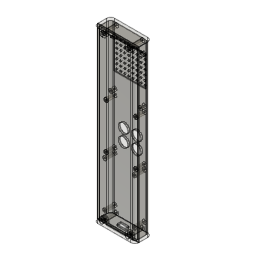
remote (Autodesk Fusion 360 design; units mm, degrees)
part number: 2025-07-19-14-33-31-747
part number: 2025-07-19-16-18-06-668
Autodesk Fusion 360 part; units mm, degrees
sketch "end" plane through (0, 0, 0) normal (0, 0, 1) x (1, 0, 0)
  line L0 (-20, 10) -> (21, 10)
  line L1 (26, 5) -> (26, -6)
  line L2 (21, -11) -> (-20, -11)
  line L3 (-25, -6) -> (-25, 5)
  arc A0 (-20, 10) -> (-25, 5) centre (-20, 5) ccw
  arc A1 (-25, -6) -> (-20, -11) centre (-20, -6) ccw
  arc A2 (26, 5) -> (21, 10) centre (21, 5) ccw
  arc A3 (21, -11) -> (26, -6) centre (21, -6) ccw
  arc A4 (24, 5) -> (21, 8) centre (21, 5) ccw
  line L4 (-20, 8) -> (21, 8)
  arc A5 (-20, 8) -> (-23, 5) centre (-20, 5) ccw
  line L5 (-23, -6) -> (-23, 5)
  arc A6 (-23, -6) -> (-20, -9) centre (-20, -6) ccw
  line L6 (21, -9) -> (-20, -9)
  arc A7 (21, -9) -> (24, -6) centre (21, -6) ccw
  line L7 (24, 5) -> (24, -6)
  point P0 (-25, 10)
  point P1 (26, 10)
  point P2 (-25, -11)
  dimension "d1" = 51
  dimension "d2" = 21
  dimension "d3" = 5
  dimension "d4" = 5
  dimension "d5" = 5
  dimension "d6" = 5
  dimension "d7" = 2
  constraint horizontal L0
  constraint vertical L1
  constraint horizontal L2
  constraint vertical L3
  constraint coincident P0 L0
  constraint coincident P0 L3
  constraint tangent L0 A0
  constraint tangent L3 A0
  constraint coincident P2 L2
  constraint coincident P2 L3
  constraint tangent L2 A1
  constraint tangent L3 A1
  constraint coincident P1 L0
  constraint coincident P1 L1
  constraint tangent L0 A2
  constraint tangent L1 A2
  constraint tangent L1 A3
  constraint tangent L2 A3
  measures "d1" distance of P0 P1
  measures "d2" distance of P0 P2
  measures "d3" radius of A0 P2
  measures "d4" radius of A1 P2
  measures "d5" radius of A2
  measures "d6" radius of A3
extrude "Extrude1" add sketch "end" along normal blind 202 makes body 1
sketch "wall" plane through (0, 0, 0) normal (0, 0, 1) x (1, 0, 0)
  line L0 (21, -11) -> (-20, -11)
  arc A0 (-20, 10) -> (-25, 5) centre (-20, 5) ccw
  line L1 (-20, 10) -> (21, 10)
  arc A1 (-25, -6) -> (-20, -11) centre (-20, -6) ccw
  line L2 (-25, -6) -> (-25, 5)
  arc A2 (21, -11) -> (26, -6) centre (21, -6) ccw
  arc A3 (26, 5) -> (21, 10) centre (21, 5) ccw
  line L3 (26, 5) -> (26, -6)
  point P0 (26, 10)
  point P1 (-25, 10)
  point P2 (-25, -11)
  dimension "d10" = 51
  dimension "d11" = 21
  dimension "d12" = 5
  dimension "d13" = 5
  dimension "d14" = 5
  dimension "d15" = 5
  constraint horizontal L1
  constraint vertical L3
  constraint horizontal L0
  constraint vertical L2
  constraint coincident P1 L1
  constraint coincident P1 L2
  constraint tangent A0 L1
  constraint tangent A0 L2
  constraint coincident P2 L0
  constraint coincident P2 L2
  constraint tangent L0 A1
  constraint tangent A1 L2
  constraint coincident P0 L1
  constraint coincident P0 L3
  constraint tangent L1 A3
  constraint tangent A3 L3
  constraint tangent A2 L3
  constraint tangent L0 A2
  measures "d10" distance of P0 P1
  measures "d11" distance of P1 P2
  measures "d12" radius of A0
  measures "d13" radius of A1
  measures "d14" radius of A3
  measures "d15" radius of A2
extrude "Extrude2" add sketch "end" along normal blind 2 separate body contours L0 L1 L2 L3 A0 A1 A2 A3 | A4 L4 A5 L5 A6 L6 A7 L7 makes body 2
copy_body "CopyPasteBodies1" bodies 2 makes body 3
move_body "Move1" bodies 3 to x (1, 0, 0) y (0, 1, 0) z (0, 0, 1) at (0, 0, 200)
cylinder "CylinderPrimitive3" add diameter 5 height 12.5 placed x (1, 0, 0) y (0, 0, -1) z (0, 1, 0) at (-55, 0, 80) separate body makes body 4
cylinder "CylinderPrimitive4" cut diameter 1.7 height -12.5 placed x (1, 0, 0) y (0, 0, 1) z (0, -1, 0) at (-55, 0, 80) bodies 4
move_body "Move2" bodies 4 to x (1, 0, 0) y (0, 1, 0) z (0, 0, 1) at (0, -4.5, 0)
move_body "Move3" bodies 4 to x (1, 0, 0) y (0, 1, 0) z (0, 0, 1) at (0, 0, -77.5)
move_body "Move4" bodies 4 to x (1, 0, 0) y (0, 1, 0) z (0, 0, 1) at (0, 0, 9.5)
move_body "Move5" bodies 4 to x (1, 0, 0) y (0, 1, 0) z (0, 0, 1) at (32.5, 0, 0)
copy_body "CopyPasteBodies2" bodies 4 makes body 5
move_body "Move6" bodies 5 to x (1, 0, 0) y (0, 1, 0) z (0, 0, 1) at (46, 0, 0)
move_body "Move7" bodies 4 to x (1, 0, 0) y (0, 1, 0) z (0, 0, 1) at (4.75, 0, 0)
move_body "Move8" bodies 5 to x (1, 0, 0) y (0, 1, 0) z (0, 0, 1) at (-4.75, 0, 0)
copy_body "CopyPasteBodies3" bodies 4 makes body 6
move_body "Move9" bodies 6 to x (1, 0, 0) y (0, 1, 0) z (0, 0, 1) at (0, 0, 56)
copy_body "CopyPasteBodies4" bodies 5 makes body 7
move_body "Move10" bodies 7 to x (1, 0, 0) y (0, 1, 0) z (0, 0, 1) at (0, 0, 56)
cylinder "CylinderPrimitive5" add diameter 5 height 10.2 placed x (1, 0, 0) y (0, 0, -1) z (0, 1, 0) at (50, 10, 10) separate body makes body 8
cylinder "CylinderPrimitive6" cut diameter 1.7 height 10.2 placed x (1, 0, 0) y (0, 0, -1) z (0, 1, 0) at (50, 10, 10) bodies 8
move_body "Move11" bodies 8 to x (1, 0, 0) y (0, 1, 0) z (0, 0, 1) at (-26.5, 0, 0)
move_body "Move12" bodies 8 to x (1, 0, 0) y (0, 1, 0) z (0, 0, 1) at (0, -12.2, 0)
copy_body "CopyPasteBodies5" bodies 8 makes body 9
move_body "Move13" bodies 9 to x (1, 0, 0) y (0, 1, 0) z (0, 0, 1) at (-46, 0, 0)
move_body "Move14" bodies 8 to x (1, 0, 0) y (0, 1, 0) z (0, 0, 1) at (-4.7, 0, 0)
move_body "Move15" bodies 9 to x (1, 0, 0) y (0, 1, 0) z (0, 0, 1) at (4.7, 0, 0)
move_body "Move16" bodies 8 9 to x (1, 0, 0) y (0, 1, 0) z (0, 0, 1) at (0, 0, -7.5)
move_body "Move17" bodies 8 9 to x (1, 0, 0) y (0, 1, 0) z (0, 0, 1) at (0, 0, 71.2)
copy_body "CopyPasteBodies6" bodies 8 9 makes body 10 makes body 11
move_body "Move18" bodies 10 11 to x (1, 0, 0) y (0, 1, 0) z (0, 0, 1) at (0, 0, 56)
cylinder "CylinderPrimitive7" add diameter 5 height 5 placed x (1, 0, 0) y (0, 0, -1) z (0, 1, 0) at (35, 0, 115) separate body makes body 12
cylinder "CylinderPrimitive8" cut diameter 1.7 height 5 placed x (1, 0, 0) y (0, 0, -1) z (0, 1, 0) at (35, 0, 115) bodies 12
move_body "Move19" bodies 12 to x (1, 0, 0) y (0, 1, 0) z (0, 0, 1) at (-11.5, 0, 84.5)
copy_body "CopyPasteBodies7" bodies 12 makes body 13
move_body "Move20" bodies 13 to x (1, 0, 0) y (0, 1, 0) z (0, 0, 1) at (-46, 0, 0)
move_body "Move21" bodies 12 to x (1, 0, 0) y (0, 1, 0) z (0, 0, 1) at (-4.7, 0, 0)
move_body "Move22" bodies 13 to x (1, 0, 0) y (0, 1, 0) z (0, 0, 1) at (4.7, 0, 0)
move_body "Move23" bodies 12 13 to x (1, 0, 0) y (0, 1, 0) z (0, 0, 1) at (0, 0, -7.1)
copy_body "CopyPasteBodies8" bodies 12 13 makes body 14 makes body 15
move_body "Move24" bodies 14 15 to x (1, 0, 0) y (0, 1, 0) z (0, 0, 1) at (0, 0, -56)
move_body "Move25" bodies 12 13 14 15 to x (1, 0, 0) y (0, 1, 0) z (0, 0, 1) at (0, 3, 0)
ref_plane "WorkPlane1" through (0, -6, 0) normal (0, 1, 0) x (0, 0, 1)
combine "Combine1" operation add target body 1 tool bodies 3 5 2 4 7 6 9 8 10 12 11 13 14 15 keep tools result as body 16 in component "Component"
split "Split1" by plane through (0, -6, 0) normal (0, 1, 0) bodies 16 makes body 17 at (-6.3333, 10, 134.6667) in component "Component"
cylinder "CylinderPrimitive9" add diameter 5 height 14 placed x (1, 0, 0) y (0, 0, -1) z (0, 1, 0) at (50, 0, 50) separate body makes body 18
cylinder "CylinderPrimitive10" cut diameter 1.7 height 14 placed x (1, 0, 0) y (0, 0, -1) z (0, 1, 0) at (50, 0, 50) bodies 18
move_body "Move26" bodies 18 to x (1, 0, 0) y (0, 1, 0) z (0, 0, 1) at (-26.5, 0, 0)
move_body "Move27" bodies 18 to x (1, 0, 0) y (0, 1, 0) z (0, 0, 1) at (0, 0, -47.5)
copy_body "CopyPasteBodies9" bodies 18 makes body 19
move_body "Move28" bodies 19 to x (1, 0, 0) y (0, 1, 0) z (0, 0, 1) at (-46, 0, 0)
move_body "Move29" bodies 18 to x (1, 0, 0) y (0, 1, 0) z (0, 0, 1) at (-7, 0, 2)
move_body "Move30" bodies 19 to x (1, 0, 0) y (0, 1, 0) z (0, 0, 1) at (7, 0, 2)
move_body "Move31" bodies 18 19 to x (1, 0, 0) y (0, 1, 0) z (0, 0, 1) at (0, -6, 0)
move_body "Move32" bodies 18 19 to x (1, 0, 0) y (0, 1, 0) z (0, 0, 1) at (0, 0, 193)
combine "Combine2" operation add target body 17 tool bodies 18 19 keep tools in component "Component"
cylinder "CylinderPrimitive11" add diameter 5 height 5 placed x (1, 0, 0) y (0, 0, -1) z (0, 1, 0) at (35, 0, 165) separate body makes body 20
move_body "Move33" bodies 20 to x (1, 0, 0) y (0, 1, 0) z (0, 0, 1) at (0, -12, 32.5)
move_body "Move34" bodies 20 to x (1, 0, 0) y (0, 1, 0) z (0, 0, 1) at (-50.5, 0, 0)
combine "Combine3" operation cut target body 16 tool bodies 20 keep tools in component "Component"
move_body "Move35" bodies 20 to x (1, 0, 0) y (0, 1, 0) z (0, 0, 1) at (32, 0, 0)
combine "Combine4" operation cut target body 16 tool bodies 20 keep tools in component "Component"
move_body "Move36" bodies 20 to x (1, 0, 0) y (0, 1, 0) z (0, 0, 1) at (0, 0, -193)
copy_body "CopyPasteBodies10" bodies 18 19 makes body 21 makes body 22
move_body "Move37" bodies 21 22 to x (1, 0, 0) y (0, 1, 0) z (0, 0, 1) at (0, 0, -193)
combine "Combine5" operation add target body 17 tool bodies 21 22 keep tools in component "Component"
combine "Combine6" operation cut target body 16 tool bodies 20 keep tools in component "Component"
move_body "Move38" bodies 20 to x (1, 0, 0) y (0, 1, 0) z (0, 0, 1) at (-32, 0, 0)
combine "Combine7" operation cut target body 16 tool bodies 20 keep tools in component "Component"
cylinder "CylinderPrimitive12" add diameter 9 height 5 placed x (1, 0, 0) y (0, 0, -1) z (0, 1, 0) at (40, 0, 5) separate body makes body 23
cylinder "CylinderPrimitive13" add diameter 5 height 3 placed x (1, 0, 0) y (0, 0, -1) z (0, 1, 0) at (40, 0, 15) separate body makes body 24
move_body "Move39" bodies 24 to x (1, 0, 0) y (0, 1, 0) z (0, 0, 1) at (0, 0, -10)
combine "Combine1'" operation cut target body 23 tool bodies 24
cylinder "CylinderPrimitive14" add diameter 2 height 5 placed x (1, 0, 0) y (0, 0, -1) z (0, 1, 0) at (50, 0, 5) separate body makes body 25
move_body "Move40" bodies 25 to x (1, 0, 0) y (0, 1, 0) z (0, 0, 1) at (-10, 0, 0)
combine "Combine2'" operation cut target body 23 tool bodies 25
move_body "Move41" bodies 23 to x (1, 0, 0) y (0, 1, 0) z (0, 0, 1) at (-23.5, -11, 0)
move_body "Move42" bodies 23 to x (1, 0, 0) y (0, 1, 0) z (0, 0, 1) at (0, 0, -0.5)
copy_body "CopyPasteBodies11" bodies 23 makes body 26
move_body "Move43" bodies 26 to x (1, 0, 0) y (0, 1, 0) z (0, 0, 1) at (-32, 0, 0)
copy_body "CopyPasteBodies12" bodies 23 26 makes body 27 makes body 28
move_body "Move44" bodies 27 28 to x (1, 0, 0) y (0, 1, 0) z (0, 0, 1) at (0, 0, 193)
combine "Combine8" operation add target body 16 tool bodies 23 26 27 28 keep tools in component "Component"
cylinder "CylinderPrimitive15" add diameter 12 height 3 placed x (1, 0, 0) y (0, 0, -1) z (0, 1, 0) at (-50, 0, 50) separate body makes body 29
move_body "Move45" bodies 29 to x (1, 0, 0) y (0, 1, 0) z (0, 0, 1) at (0, 7.5, 0)
move_body "Move46" bodies 29 to x (1, 0, 0) y (0, 1, 0) z (0, 0, 1) at (70, 0, 34)
move_body "Move47" bodies 29 to x (1, 0, 0) y (0, 1, 0) z (0, 0, 1) at (-11.5, 0, 0)
copy_body "CopyPasteBodies13" bodies 29 makes body 30
move_body "Move48" bodies 30 to x (1, 0, 0) y (0, 1, 0) z (0, 0, 1) at (-27.5, 0, 0)
move_body "Move49" bodies 30 to x (1, 0, 0) y (0, 1, 0) z (0, 0, 1) at (11.5, 0, 0)
copy_body "CopyPasteBodies14" bodies 29 30 makes body 31 makes body 32
move_body "Move50" bodies 31 32 to x (1, 0, 0) y (0, 1, 0) z (0, 0, 1) at (0, 0, 14.8)
combine "Combine9" operation cut target body 17 tool bodies 29 30 31 32 keep tools in component "Component"
cylinder "CylinderPrimitive16" add diameter 2 height 5 placed x (1, 0, 0) y (0, 0, -1) z (0, 1, 0) at (82.0481, 0, 56.4909) separate body makes body 33
pattern_linear "R-Pattern1" count 8 spacing 5 along (1, 0, 0) count 10 spacing 5.5556 along (0, 0, 1) of bodies 33 makes body 34 at (87.9878, 1.6667, 56.1489) makes body 35 at (92.9878, 1.6667, 56.1489) makes body 36 at (97.9878, 1.6667, 56.1489) makes body 37 at (102.9878, 1.6667, 56.1489) makes body 38 at (107.9878, 1.6667, 56.1489) makes body 39 at (112.9878, 1.6667, 56.1489) makes body 40 at (117.9878, 1.6667, 56.1489) makes body 41 at (82.9878, 1.6667, 61.7044) makes body 42 at (87.9878, 1.6667, 61.7044) makes body 43 at (92.9878, 1.6667, 61.7044) makes body 44 at (97.9878, 1.6667, 61.7044) makes body 45 at (102.9878, 1.6667, 61.7044) makes body 46 at (107.9878, 1.6667, 61.7044) makes body 47 at (112.9878, 1.6667, 61.7044) makes body 48 at (117.9878, 1.6667, 61.7044) makes body 49 at (81.079, 1.6667, 67.3552) makes body 50 at (86.079, 1.6667, 67.3552) makes body 51 at (91.079, 1.6667, 67.3552) makes body 52 at (96.079, 1.6667, 67.3552) makes body 53 at (101.079, 1.6667, 67.3552) makes body 54 at (106.079, 1.6667, 67.3552) makes body 55 at (111.079, 1.6667, 67.3552) makes body 56 at (116.079, 1.6667, 67.3552) makes body 57 at (81.079, 1.6667, 72.9108) makes body 58 at (86.079, 1.6667, 72.9108) makes body 59 at (91.079, 1.6667, 72.9108) makes body 60 at (96.079, 1.6667, 72.9108) makes body 61 at (101.079, 1.6667, 72.9108) makes body 62 at (106.079, 1.6667, 72.9108) makes body 63 at (111.079, 1.6667, 72.9108) makes body 64 at (116.079, 1.6667, 72.9108) makes body 65 at (81.079, 1.6667, 78.4663) makes body 66 at (86.079, 1.6667, 78.4663) makes body 67 at (91.079, 1.6667, 78.4663) makes body 68 at (96.079, 1.6667, 78.4663) makes body 69 at (101.079, 1.6667, 78.4663) makes body 70 at (106.079, 1.6667, 78.4663) makes body 71 at (111.079, 1.6667, 78.4663) makes body 72 at (116.079, 1.6667, 78.4663) makes body 73 at (81.079, 1.6667, 84.0219) makes body 74 at (86.079, 1.6667, 84.0219) makes body 75 at (91.079, 1.6667, 84.0219) makes body 76 at (96.079, 1.6667, 84.0219) makes body 77 at (101.079, 1.6667, 84.0219) makes body 78 at (106.079, 1.6667, 84.0219) makes body 79 at (111.079, 1.6667, 84.0219) makes body 80 at (116.079, 1.6667, 84.0219) makes body 81 at (81.079, 1.6667, 89.5775) makes body 82 at (86.079, 1.6667, 89.5775) makes body 83 at (91.079, 1.6667, 89.5775) makes body 84 at (96.079, 1.6667, 89.5775) makes body 85 at (101.079, 1.6667, 89.5775) makes body 86 at (106.079, 1.6667, 89.5775) makes body 87 at (111.079, 1.6667, 89.5775) makes body 88 at (116.079, 1.6667, 89.5775) makes body 89 at (81.079, 1.6667, 95.133) makes body 90 at (86.079, 1.6667, 95.133) makes body 91 at (91.079, 1.6667, 95.133) makes body 92 at (96.079, 1.6667, 95.133) makes body 93 at (101.079, 1.6667, 95.133) makes body 94 at (106.079, 1.6667, 95.133) makes body 95 at (111.079, 1.6667, 95.133) makes body 96 at (116.079, 1.6667, 95.133) makes body 97 at (81.079, 1.6667, 100.6886) makes body 98 at (86.079, 1.6667, 100.6886) makes body 99 at (91.079, 1.6667, 100.6886) makes body 100 at (96.079, 1.6667, 100.6886) makes body 101 at (101.079, 1.6667, 100.6886) makes body 102 at (106.079, 1.6667, 100.6886) makes body 103 at (111.079, 1.6667, 100.6886) makes body 104 at (116.079, 1.6667, 100.6886) makes body 105 at (81.079, 1.6667, 106.2441) makes body 106 at (86.079, 1.6667, 106.2441) makes body 107 at (91.079, 1.6667, 106.2441) makes body 108 at (96.079, 1.6667, 106.2441) makes body 109 at (101.079, 1.6667, 106.2441) makes body 110 at (106.079, 1.6667, 106.2441) makes body 111 at (111.079, 1.6667, 106.2441) makes body 112 at (116.079, 1.6667, 106.2441)
move_body "Move51" bodies 104 91 66 34 101 65 38 82 85 81 67 48 41 108 59 86 70 106 89 39 61 57 79 77 96 75 102 71 98 109 78 99 36 95 83 37 111 80 69 110 53 44 33 103 49 112 84 58 43 52 51 45 76 50 42 62 88 100 107 105 40 46 73 64 97 47 92 72 55 54 87 35 63 93 68 56 74 94 60 90 to x (1, 0, 0) y (0, 1, 0) z (0, 0, 1) at (-99, 0, 84)
move_body "Move52" bodies 33 58 60 59 61 62 63 56 57 55 35 34 71 70 72 73 74 75 65 67 64 66 68 69 48 46 47 52 54 53 38 37 44 45 43 36 94 95 96 98 97 99 101 100 102 103 104 105 42 79 81 80 82 83 84 85 88 86 87 90 89 93 91 92 77 78 76 40 41 39 50 51 49 107 108 106 109 111 110 112 to x (1, 0, 0) y (0, 1, 0) z (0, 0, 1) at (0, -12, 0)
combine "Combine10" operation cut target body 17 tool bodies 33 58 60 59 61 62 63 56 57 55 35 34 71 70 72 73 74 75 65 67 64 66 68 69 48 46 47 52 54 53 38 37 44 45 43 36 94 95 96 98 97 99 101 100 102 103 104 105 42 79 81 80 82 83 84 85 88 86 87 90 89 93 91 92 77 78 76 40 41 39 50 51 49 107 108 106 109 111 110 112 keep tools in component "Component"
move_body "Move53" bodies 34 46 90 60 61 96 79 38 36 56 111 97 99 104 81 92 43 109 103 83 95 40 89 100 42 45 67 107 35 48 39 84 33 91 112 106 50 57 74 108 53 88 44 64 75 63 73 59 87 47 52 76 78 71 65 70 77 49 105 72 69 80 101 102 85 93 110 62 41 68 94 54 82 37 66 51 98 55 58 86 to x (1, 0, 0) y (0, 1, 0) z (0, 0, 1) at (0, 19, 0)
combine "Combine11" operation cut target body 17 tool bodies 33 58 60 59 61 62 63 56 57 55 35 34 71 70 72 73 74 75 65 67 64 66 68 69 48 46 47 52 54 53 38 37 44 45 43 36 94 95 96 98 97 99 101 100 102 103 104 105 42 79 81 80 82 83 84 85 88 86 87 90 89 93 91 92 77 78 76 40 41 39 50 51 49 107 108 106 109 111 110 112 keep tools in component "Component"
box "BoxPrimitive1" add length 5 width 10 height 4 placed x (0, 1, 0) y (-1, 0, 0) z (0, 0, 1) at (-1, 21, 0) separate body makes body 113
move_body "Move54" bodies 113 to x (1, 0, 0) y (0, 1, 0) z (0, 0, 1) at (0, -16, 0)
move_body "Move55" bodies 113 to x (1, 0, 0) y (0, 1, 0) z (0, 0, 1) at (-14, -6.5, 0)
move_body "Move56" bodies 113 to x (1, 0, 0) y (0, 1, 0) z (0, 0, 1) at (20.5, 0, 0)
move_body "Move57" bodies 113 to x (1, 0, 0) y (0, 1, 0) z (0, 0, 1) at (-1.27, 0, 0)
combine "Combine12" operation cut target body 17 tool bodies 113 keep tools in component "Component"
box "BoxPrimitive2" add length 6 width 43 height 2 placed x (0, 0, -1) y (-1, 0, 0) z (0, 1, 0) at (22, 0, 195) separate body makes body 114
move_body "Move58" bodies 114 to x (1, 0, 0) y (0, 1, 0) z (0, 0, 1) at (0, 3, 0)
combine "Combine13" operation cut target body 17 tool bodies 114 keep tools in component "Component"
cylinder "CylinderPrimitive17" add diameter 5 height 2 placed x (1, 0, 0) y (0, 0, -1) z (0, 1, 0) at (-15, 10, 130) separate body makes body 115
move_body "Move59" bodies 115 to x (1, 0, 0) y (0, 1, 0) z (0, 0, 1) at (-2.8, 0, -0.3)
cylinder "CylinderPrimitive18" add diameter 1.7 height 2 placed x (1, 0, 0) y (0, 0, -1) z (0, 1, 0) at (-20, 10, 139) separate body makes body 116
move_body "Move60" bodies 116 to x (1, 0, 0) y (0, 1, 0) z (0, 0, 1) at (2.2, 0, -2.6)
move_body "Move61" bodies 116 to x (1, 0, 0) y (0, 1, 0) z (0, 0, 1) at (0, 0, -6.7)
move_body "Move62" bodies 116 to x (1, 0, 0) y (0, 1, 0) z (0, 0, 1) at (0, -12.2, 0)
move_body "Move63" bodies 115 to x (1, 0, 0) y (0, 1, 0) z (0, 0, 1) at (0, -14.2, 0)
move_body "Move64" bodies 116 to x (1, 0, 0) y (0, 1, 0) z (0, 0, 1) at (0, -2, 0)
combine "Combine3'" operation cut target body 115 tool bodies 116
combine "Combine14" operation add target body 17 tool bodies 115 keep tools in component "Component"
scale "Scale1" factors (1, 2, 1) about (-16.95, -4.2, 129.7) bodies 115
combine "Combine15" operation add target body 17 tool bodies 115 keep tools in component "Component"
box "BoxPrimitive4" add length 16 width 39 height 2 placed x (0, 0, -1) y (-1, 0, 0) z (0, 1, 0) at (20, 10, 155) separate body makes body 117
move_body "Move69" bodies 117 to x (1, 0, 0) y (0, 1, 0) z (0, 0, 1) at (0, -2, 0)
combine "Combine20" operation add target body 17 tool bodies 117 in component "Component"
cylinder "CylinderPrimitive19" add diameter 5 height 3 placed x (1, 0, 0) y (0, 0, -1) z (0, 1, 0) at (35, 0, 185) separate body makes body 118
move_body "Move70" bodies 118 to x (1, 0, 0) y (0, 1, 0) z (0, 0, 1) at (-2.7791, 5, 7.5018)
move_body "Move71" bodies 118 to x (1, 0, 0) y (0, 1, 0) z (0, 0, 1) at (-13.4, 0, -0.1)
combine "Combine21" operation add target body 17 tool bodies 118 keep tools in component "Component"
move_body "Move72" bodies 118 to x (1, 0, 0) y (0, 1, 0) z (0, 0, 1) at (-36.6, 0, 0)
combine "Combine22" operation add target body 17 tool bodies 118 in component "Component"
box "BoxPrimitive5" add length 8 width 41 height 2 placed x (0, 0, 1) y (1, 0, 0) z (0, 1, 0) at (-20, 0, 184) separate body makes body 119
move_body "Move73" bodies 119 to x (1, 0, 0) y (0, 1, 0) z (0, 0, 1) at (0, 6, 0)
scale "Scale2" factors (1, 1.5, 1) about (-20, 8, 192) bodies 119
combine "Combine23" operation cut target body 17 tool bodies 119 in component "Component"
box "BoxPrimitive6" add length 37 width 39 height 1 placed x (0, 0, 1) y (-1, 0, 0) z (0, -1, 0) at (20, 8, 155) separate body makes body 120
move_body "Move74" bodies 120 to x (1, 0, 0) y (0, 1, 0) z (0, 0, 1) at (0, 1, 0)
combine "Combine24" operation cut target body 17 tool bodies 120 in component "Component"
box "BoxPrimitive7" add length 7 width 7 height 3 placed x (0, 0, 1) y (1, 0, 0) z (0, 1, 0) at (-21, 10, 133) separate body makes body 121
move_body "Move75" bodies 121 to x (1, 0, 0) y (0, 1, 0) z (0, 0, 1) at (0, -15.2, -7)
combine "Combine25" operation cut target body 17 tool bodies 121 in component "Component"
cylinder "CylinderPrimitive20" add diameter 5 height 1 placed x (1, 0, 0) y (0, 0, -1) z (0, 1, 0) at (35, 0, 70) separate body makes body 122
cylinder "CylinderPrimitive21" cut diameter 1.7 height 1 placed x (1, 0, 0) y (0, 0, -1) z (0, 1, 0) at (35, 0, 70) bodies 122
move_body "Move76" bodies 122 to x (1, 0, 0) y (0, 1, 0) z (0, 0, 1) at (-16.2, 0, 3.7)
move_body "Move77" bodies 122 to x (1, 0, 0) y (0, 1, 0) z (0, 0, 1) at (0, -3.2, 0)
combine "Combine26" operation add target body 17 tool bodies 122 keep tools in component "Component"
move_body "Move78" bodies 122 to x (1, 0, 0) y (0, 1, 0) z (0, 0, 1) at (-36.6, 0, 0)
combine "Combine27" operation add target body 17 tool bodies 122 keep tools in component "Component"
move_body "Move79" bodies 122 to x (1, 0, 0) y (0, 1, 0) z (0, 0, 1) at (0, 0, 56)
combine "Combine28" operation add target body 17 tool bodies 122 keep tools in component "Component"
move_body "Move80" bodies 122 to x (1, 0, 0) y (0, 1, 0) z (0, 0, 1) at (36.6, 0, 0)
combine "Combine29" operation add target body 17 tool bodies 122 in component "Component"
ref_plane "WorkPlane2" through (0, 0, 195) normal (0, 0, 1) x (1, 0, 0)
split "Split2" by plane through (0, 0, 195) normal (0, 0, 1) bodies 17 makes body 123 at (7.3333, -0.6667, 202) in component "Component"
split "Split3" by plane through (0, 0, 195) normal (0, 0, 1) bodies 16 makes body 124 at (-3.3494, -11, 197.2603) in component "Component"
move_body "Move1'" bodies 123 to x (1, 0, 0) y (0, 1, 0) z (0, 0, 1) at (0, 0, 8) in component "Component"
move_body "Move2'" bodies 124 to x (1, 0, 0) y (0, 1, 0) z (0, 0, 1) at (0, 0, 8) in component "Component"
ref_plane "WorkPlane3" through (0, 0, 115) normal (0, 0, 1) x (1, 0, 0)
ref_plane "WorkPlane4" through (0, 0, 107) normal (0, 0, 1) x (1, 0, 0)
split "Split4" by plane through (0, 0, 115) normal (0, 0, 1) bodies 17 makes body 125 at (-0.2726, 10, 128.7222) in component "Component"
split "Split5" by plane through (0, 0, 115) normal (0, 0, 1) bodies 16 makes body 126 at (-4.4181, -11, 141.0586) in component "Component"
split "Split6" by plane through (0, 0, 107) normal (0, 0, 1) bodies 17 makes body 127 at (-6.3333, 8, 112.3333) in component "Component"
split "Split7" by plane through (0, 0, 107) normal (0, 0, 1) bodies 16 makes body 128 at (7.3333, -11, 112.3333) in component "Component"
copy_body "CopyPasteBodies15" bodies 127 makes body 129
move_body "Move81" bodies 129 to x (1, 0, 0) y (0, 1, 0) z (0, 0, 1) at (0, 0, 88)
copy_body "CopyPasteBodies16" bodies 128 makes body 130
move_body "Move82" bodies 130 to x (1, 0, 0) y (0, 1, 0) z (0, 0, 1) at (0, 0, 88)
combine "Combine30" operation add target body 17 tool bodies 123 125 127 129 in component "Component"
combine "Combine31" operation add target body 16 tool bodies 124 126 128 130 in component "Component"
ref_plane "WorkPlane5" through (0, 0, 190) normal (0, 0, 1) x (1, 0, 0)
ref_plane "WorkPlane6" through (0, 0, 203) normal (0, 0, 1) x (1, 0, 0)
ref_plane "WorkPlane7" through (0, 0, 198) normal (0, 0, 1) x (1, 0, 0)
split "Split8" by plane through (0, 0, 203) normal (0, 0, 1) bodies 16 makes body 131 at (-3.3494, -11, 205.2603) in component "Component"
split "Split9" by plane through (0, 0, 198) normal (0, 0, 1) bodies 16 makes body 132 at (-3.5861, -11, 199.6667) in component "Component"
split "Split10" by plane through (0, 0, 190) normal (0, 0, 1) bodies 16 makes body 133 at (5.4181, -11, 191.0586) in component "Component"
split "Split11" by plane through (0, 0, 195) normal (0, 0, 1) bodies 133 makes body 134 at (-3.5861, -9, 197) in component "Component"
move_body "Move3'" bodies 132 to x (1, 0, 0) y (0, 1, 0) z (0, 0, 1) at (0, 0, -8) in component "Component"
move_body "Move4'" bodies 133 to x (1, 0, 0) y (0, 1, 0) z (0, 0, 1) at (0, 0, 8) in component "Component"
combine "Combine32" operation add target body 16 tool bodies 131 132 133 134 in component "Component"
move_body "Move65" [suppressed]
combine "Combine16" [suppressed] in component "Component"
move_body "Move66" [suppressed]
combine "Combine17" [suppressed] in component "Component"
move_body "Move67" [suppressed]
combine "Combine18" [suppressed] in component "Component"
boxprimitive "BoxPrimitive3" [suppressed]
move_body "Move68" [suppressed]
combine "Combine19" [suppressed] in component "Component"
component "Component" placed x (1, 0, 0) y (0, 1, 0) z (0, 0, 1) at (0, 0, 0)
hidden bodies 1 2 3 4 5 6 7 8 9 10 11 12 13 14 15 18 19 21 22 20 23 26 27 28 29 30 31 32 33 34 35 36 37 38 39 40 41 42 43 44 45 46 47 48 49 50 51 52 53 54 55 56 57 58 59 60 61 62 63 64 65 66 67 68 69 70 71 72 73 74 75 76 77 78 79 80 81 82 83 84 85 86 87 88 89 90 91 92 93 94 95 96 97 98 99 100 101 102 103 104 105 106 107 108 109 110 111 112 113 114 115
named bodies: "Wall", "port_end", "light_end", "huzzah_spacer_1", "huzzah_spacer_2", "huzzah_spacer_1 (1)", "huzzah_spacer_3", "huzzah_spacer_4", "button_spacer_1", "button_spacer_2", "button_spacer_1 (1)", "button_spacer_3", "button_spacer_4", "light_spacer_1", "light_spacer_2", "light_spacer_1 (1)", "light_spacer_3", "light_spacer_4", "bottom", "top", "remote_spacer_1", "remote_spacer_2", "remote_spacer_1 (1)", "remote_spacer_3", "remote_spacer_4", "screw_socket_1", "screw_socket_2", "screw_socket_1 (1)", "screw_socket_3", "screw_socket_4", "button_hole_1", "button_hole_2", "button_hole_3", "button_hole_4", "top (1)", "bottom (1)", "top (2)", "bottom (2)", "top (3)", "bottom (3)", "bottom (3) (1)"
